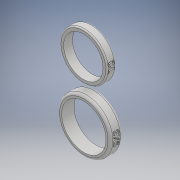
# Autodesk Inventor part: Rings
Saved by Autodesk Inventor 2018 (Build 220112000, 112)
## iProperties
Created: 2021-07-04
Part Number: Rings
Material: Generic
Document SubType Name: Modeling
Designer: dangl
Density: 1 g/cm^3
Appearance: Default
Author: dangl
Autodesk Inventor part; units mm, degrees
note: some values were not read from the file. Chosen so that the rebuilt part matches the saved one: direction of "Emboss1"; direction of "Emboss2".
ref_plane "XZ Plane" through (0, 0, 0) normal (0, 1, 0) x (-1, 0, 0)
ref_plane "XY Plane" through (0, 0, 0) normal (0, 0, 1) x (1, 0, 0)
sketch "Sketch1" plane through (0, 0, 0) normal (0, 1, 0) x (-1, 0, 0)
  circle A0 centre (0, 0) radius 9
  circle A1 centre (0.2028, 24.5776) radius 8
  circle A2 centre (0.2028, 24.5776) radius 9.6
  circle A3 centre (0, 0) radius 10.8
  dimension "d0" = 18
  dimension "d1" = 16
  dimension "d2" = 1.6
  dimension "d3" = 1.8
  constraints: 4 centre point, 1 coincident
  measures "d0" diameter of A0
  measures "d1" diameter of A1
  measures "d2" radial gap between concentric circles of A1 A2
  measures "d3" radial gap between concentric circles of A0 A3
extrude "Extrusion1" add sketch "Sketch1" along normal blind 5 contours A3
extrude "Extrusion2" add sketch "Sketch1" along normal blind 3.6 contours A2
fillet "Fillet1" radius 0.5 2 edges at (9.3972, 3.6, 24.5776) (9.3972, 0, 24.5776)
fillet "Fillet2" radius 1 2 edges at (10.8, 0, 0) (10.8, 5, 0)
ref_plane "Work Plane1" through (14.75, 0, 0) normal (1, 0, 0) x (0, 1, 0)
sketch "Sketch2" plane through (14.75, 0, 0) normal (1, 0, 0) x (0, 1, 0)
  line L0 (2.9528, 26.9029) -> (2.9528, 22.7113) construction
  line L1 (2.9528, 22.7113) -> (-0.5176, 22.7113) construction
  line L2 (-0.5176, 22.7113) -> (-0.5176, 26.9029) construction
  line L3 (-0.5176, 26.9029) -> (2.9528, 26.9029) construction
  line L4 (3.6702, 2.9394) -> (3.6702, -1.2522) construction
  line L5 (3.6702, -1.2522) -> (0.1998, -1.2522) construction
  line L6 (0.1998, -1.2522) -> (0.1998, 2.9394) construction
  line L7 (0.1998, 2.9394) -> (3.6702, 2.9394) construction
  line L8 (0.6528, 26.6405) -> (2.9528, 26.6405)
  line L9 (2.9528, 26.6405) -> (2.9528, 25.8255)
  spline S0 degree 2 poles (2.9528, 25.8255) (2.9528, 24.5986) (1.8326, 24.5986) knots 0 0 0 1 1 1
  spline S1 degree 2 poles (1.8326, 24.5986) (1.295, 24.5986) (0.6528, 25.2686) (0.6528, 25.8255) knots 0 0 0 1 2 2 2
  line L10 (0.6528, 25.8255) -> (0.6528, 26.6405)
  line L11 (2.5324, 26.122) -> (1.0731, 26.122)
  line L12 (1.0731, 26.122) -> (1.0731, 25.8639)
  spline S2 degree 2 poles (1.0731, 25.8639) (1.0731, 25.5289) (1.4785, 25.1448) (1.8262, 25.1448) knots 0 0 0 1 2 2 2
  spline S3 degree 2 poles (1.8262, 25.1448) (2.1548, 25.1448) (2.5324, 25.5246) (2.5324, 25.8681) knots 0 0 0 1 2 2 2
  line L13 (2.5324, 25.8681) -> (2.5324, 26.122)
  line L14 (0.6528, 22.8491) -> (0.6528, 24.2189)
  line L15 (0.6528, 24.2189) -> (2.9528, 24.2189)
  line L16 (2.9528, 24.2189) -> (2.9528, 23.7004)
  line L17 (2.9528, 23.7004) -> (1.0731, 23.7004)
  line L18 (1.0731, 23.7004) -> (1.0731, 22.8491)
  line L19 (1.0731, 22.8491) -> (0.6528, 22.8491)
  line L20 (1.4192, 2.7816) -> (1.9334, 2.7816)
  spline S4 degree 2 poles (1.9334, 2.7816) (1.8161, 2.6429) (1.6987, 2.3143) (1.6987, 2.1479) knots 0 0 0 1 2 2 2
  spline S5 degree 2 poles (1.6987, 2.1479) (1.6987, 2.0497) (1.735, 1.9047) (1.7969, 1.8065) (1.8822, 1.7596) (1.9313, 1.7596) knots 0 0 0 1 2 3 4 4 4
  spline S6 degree 2 poles (1.9313, 1.7596) (1.9996, 1.7596) (2.1041, 1.8364) (2.1958, 1.9687) (2.2791, 2.1522) (2.3217, 2.2567) knots 0 0 0 1 2 3 4 4 4
  spline S7 degree 2 poles (2.3217, 2.2567) (2.4348, 2.5277) (2.757, 2.7922) (2.9874, 2.7922) knots 0 0 0 1 2 2 2
  spline S8 degree 2 poles (2.9874, 2.7922) (3.1666, 2.7922) (3.4248, 2.6471) (3.5933, 2.3996) (3.6702, 2.0711) (3.6702, 1.8876) knots 0 0 0 1 2 3 4 4 4
  spline S9 degree 2 poles (3.6702, 1.8876) (3.6702, 1.7084) (3.6275, 1.431) (3.5827, 1.3137) knots 0 0 0 1 2 2 2
  line L21 (3.5827, 1.3137) -> (3.1026, 1.3137)
  spline S10 degree 2 poles (3.1026, 1.3137) (3.1432, 1.3713) (3.205, 1.5078) (3.2434, 1.6529) (3.2626, 1.7958) (3.2626, 1.8599) knots 0 0 0 1 2 3 4 4 4
  spline S11 degree 2 poles (3.2626, 1.8599) (3.2626, 1.9473) (3.2306, 2.0924) (3.1688, 2.1927) (3.0834, 2.246) (3.0301, 2.246) knots 0 0 0 1 2 3 4 4 4
  spline S12 degree 2 poles (3.0301, 2.246) (2.9725, 2.246) (2.8807, 2.1863) (2.7997, 2.0732) (2.7207, 1.9132) (2.6802, 1.8108) knots 0 0 0 1 2 3 4 4 4
  spline S13 degree 2 poles (2.6802, 1.8108) (2.6226, 1.6742) (2.4924, 1.4545) (2.3281, 1.2966) (2.1169, 1.2134) (1.9782, 1.2134) knots 0 0 0 1 2 3 4 4 4
  spline S14 degree 2 poles (1.9782, 1.2134) (1.7862, 1.2134) (1.5238, 1.3585) (1.3616, 1.6102) (1.2912, 1.9409) (1.2912, 2.1266) knots 0 0 0 1 2 3 4 4 4
  spline S15 degree 2 poles (1.2912, 2.1266) (1.2912, 2.3143) (1.3552, 2.6578) (1.4192, 2.7816) knots 0 0 0 1 2 2 2
  line L22 (1.3317, -1.0439) -> (1.3317, -0.4295)
  line L23 (1.3317, -0.4295) -> (2.0806, -0.0326)
  spline S16 degree 2 poles (2.0806, -0.0326) (2.1233, -0.0113) (2.2343, 0.0143) knots 0 0 0 1 1 1
  line L24 (2.2343, 0.0143) -> (2.2343, 0.0207)
  spline S17 degree 2 poles (2.2343, 0.0207) (2.183, 0.0314) (2.0742, 0.0719) knots 0 0 0 1 1 1
  line L25 (2.0742, 0.0719) -> (1.3317, 0.4709)
  line L26 (1.3317, 0.4709) -> (1.3317, 1.0875)
  line L27 (1.3317, 1.0875) -> (2.4817, 0.3557)
  line L28 (2.4817, 0.3557) -> (3.6317, 1.0256)
  line L29 (3.6317, 1.0256) -> (3.6317, 0.3962)
  line L30 (3.6317, 0.3962) -> (2.9426, 0.0655)
  spline S18 degree 2 poles (2.9426, 0.0655) (2.8615, 0.0271) (2.7484, -0.0028) knots 0 0 0 1 1 1
  line L31 (2.7484, -0.0028) -> (2.7484, -0.0092)
  spline S19 degree 2 poles (2.7484, -0.0092) (2.8167, -0.0284) (2.949, -0.0817) knots 0 0 0 1 1 1
  line L32 (2.949, -0.0817) -> (3.6317, -0.4465)
  line L33 (3.6317, -0.4465) -> (3.6317, -1.0247)
  line L34 (3.6317, -1.0247) -> (2.4924, -0.3356)
  line L35 (2.4924, -0.3356) -> (1.3317, -1.0439)
  line L36 (1.4192, -1.2125) -> (1.9334, -1.2125)
  spline S20 degree 2 poles (1.9334, -1.2125) (1.8161, -1.3512) (1.6987, -1.6798) (1.6987, -1.8462) knots 0 0 0 1 2 2 2
  spline S21 degree 2 poles (1.6987, -1.8462) (1.6987, -1.9443) (1.735, -2.0894) (1.7969, -2.1875) (1.8822, -2.2345) (1.9313, -2.2345) knots 0 0 0 1 2 3 4 4 4
  spline S22 degree 2 poles (1.9313, -2.2345) (1.9996, -2.2345) (2.1041, -2.1577) (2.1958, -2.0254) (2.2791, -1.8419) (2.3217, -1.7374) knots 0 0 0 1 2 3 4 4 4
  spline S23 degree 2 poles (2.3217, -1.7374) (2.4348, -1.4664) (2.757, -1.2018) (2.9874, -1.2018) knots 0 0 0 1 2 2 2
  spline S24 degree 2 poles (2.9874, -1.2018) (3.1666, -1.2018) (3.4248, -1.3469) (3.5933, -1.5944) (3.6702, -1.923) (3.6702, -2.1065) knots 0 0 0 1 2 3 4 4 4
  spline S25 degree 2 poles (3.6702, -2.1065) (3.6702, -2.2857) (3.6275, -2.5631) (3.5827, -2.6804) knots 0 0 0 1 2 2 2
  line L37 (3.5827, -2.6804) -> (3.1026, -2.6804)
  spline S26 degree 2 poles (3.1026, -2.6804) (3.1432, -2.6228) (3.205, -2.4863) (3.2434, -2.3412) (3.2626, -2.1982) (3.2626, -2.1342) knots 0 0 0 1 2 3 4 4 4
  spline S27 degree 2 poles (3.2626, -2.1342) (3.2626, -2.0467) (3.2306, -1.9016) (3.1688, -1.8014) (3.0834, -1.748) (3.0301, -1.748) knots 0 0 0 1 2 3 4 4 4
  spline S28 degree 2 poles (3.0301, -1.748) (2.9725, -1.748) (2.8807, -1.8078) (2.7997, -1.9209) (2.7207, -2.0809) (2.6802, -2.1833) knots 0 0 0 1 2 3 4 4 4
  spline S29 degree 2 poles (2.6802, -2.1833) (2.6226, -2.3198) (2.4924, -2.5396) (2.3281, -2.6975) (2.1169, -2.7807) (1.9782, -2.7807) knots 0 0 0 1 2 3 4 4 4
  spline S30 degree 2 poles (1.9782, -2.7807) (1.7862, -2.7807) (1.5238, -2.6356) (1.3616, -2.3838) (1.2912, -2.0531) (1.2912, -1.8675) knots 0 0 0 1 2 3 4 4 4
  spline S31 degree 2 poles (1.2912, -1.8675) (1.2912, -1.6798) (1.3552, -1.3363) (1.4192, -1.2125) knots 0 0 0 1 2 2 2
  point P0 (0, 0)
  constraints: 4 other
emboss "Emboss1" sketch "Sketch2" operation cut depth 0.5 direction (-1, 0, 0) contours L8 L9 S0 S1 L10 | L14 L15 L16 L17 L18 L19
emboss "Emboss2" sketch "Sketch2" operation cut depth 0.5 direction (-1, 0, 0) contours L20 S4 S5 S6 S7 S8 S9 L21 S10 S11 S12 S13 S14 S15 | L22 L23 S16 L24 S17 L25 L26 L27 L28 L29 L30 S18 L31 S19 L32 L33 L34 L35 | L36 S20 S21 S22 S23 S24 S25 L37 S26 S27 S28 S29 S30 S31
body "Solid1"
